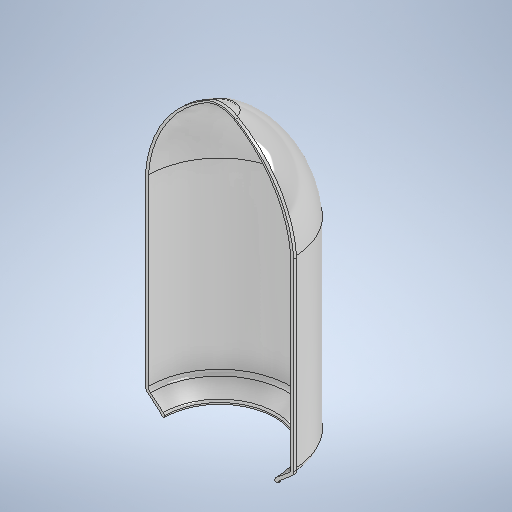
# Autodesk Inventor part: PAY-LOAD
Saved by Autodesk Inventor 2025 (Build 290162000, 162)
## iProperties
Created: 2024-07-25
Part Number: PAY-LOAD
Material: Generic
Document SubType Name: Modeling
Designer: Richard
Density: 1 g/cm^3
Appearance: Default
Author: Richard
Autodesk Inventor part; units mm, degrees
ref_plane "YZ Plane" through (0, 0, 0) normal (1, 0, 0) x (0, 1, 0)
ref_plane "XZ Plane" through (0, 0, 0) normal (0, 1, 0) x (-1, 0, 0)
ref_plane "XY Plane" through (0, 0, 0) normal (0, 0, 1) x (1, 0, 0)
sketch "Sketch1" plane through (0, 0, 0) normal (0, 0, 1) x (1, 0, 0)
  line L0 (0, 0) -> (39, 0)
  line L1 (0, 0.6011) -> (0, 0)
  line L2 (1, 1.0674) -> (1, 0)
  line L3 (39, 2) -> (39, 202)
  line L4 (-10, 138.8438) -> (-10, 13.0953)
  line L5 (0.2856, 2.5995) -> (-8.5712, 10.0311)
  line L6 (1, 2) -> (17.3022, 2) construction
  line L7 (0, 2) -> (16.6045, 2) construction
  line L8 (-6.0027, 6.5705) -> (-0.7144, 2.1332)
  line L9 (-6.0027, 6.5705) -> (-9.5712, 9.5648)
  line L10 (-11, 138.8438) -> (-11, 12.629)
  arc A0 (-10, 13.0953) -> (-8.5712, 10.0311) centre (-6, 13.0953) ccw
  arc A1 (-11, 12.629) -> (-9.5712, 9.5648) centre (-7, 12.629) ccw
  arc A2 (29, 202) -> (-11, 138.8438) centre (68.7541, 132.5766) ccw
  arc A3 (30, 202) -> (-10, 138.8438) centre (69.7541, 132.5766) ccw
  line L11 (39, 204.4115) -> (39, 205.0334)
  line L12 (39, 2) -> (39, 0)
  arc A4 (1, 1.0674) -> (0.2856, 2.5995) centre (-1, 1.0674) ccw
  arc A5 (0, 0.6011) -> (-0.7144, 2.1332) centre (-2, 0.6011) ccw
  line L13 (0, 0) -> (-1, 0)
  line L14 (-5.4284, 4.7832) -> (-10.5712, 9.0985)
  line L15 (-5.4284, 4.7832) -> (-1.7144, 1.6669)
  line L16 (-1, 0) -> (-1, 0.1348)
  line L17 (-11, 138.8438) -> (-12, 138.8438)
  line L18 (-12, 138.8438) -> (-12, 12.1627)
  arc A6 (-12, 12.1627) -> (-10.5712, 9.0985) centre (-8, 12.1627) ccw
  arc A7 (-1, 0.1348) -> (-1.7144, 1.6669) centre (-3, 0.1348) ccw
  arc A8 (28, 202) -> (-12, 138.8438) centre (67.7541, 132.5766) ccw
  arc A9 (39, 205.2967) -> (28, 202) centre (39, 185.2967) ccw
  arc A10 (39, 204.6795) -> (29, 202) centre (39, 184.6795) ccw
  arc A11 (39, 204.1394) -> (30, 202) centre (39, 184.1394) ccw
  line L19 (39, 204.1394) -> (39, 205.2967)
  line L20 (78, 0.6011) -> (78, 0)
  line L21 (84.0027, 6.5705) -> (78.7144, 2.1332)
  line L22 (84.0027, 6.5705) -> (87.5712, 9.5648)
  line L23 (89, 138.8438) -> (89, 12.629)
  arc A12 (87.5712, 9.5648) -> (89, 12.629) centre (85, 12.629) ccw
  arc A13 (89, 138.8438) -> (49, 202) centre (9.2459, 132.5766) ccw
  arc A14 (78.7144, 2.1332) -> (78, 0.6011) centre (80, 0.6011) ccw
  line L24 (78, 0) -> (79, 0)
  line L25 (83.4284, 4.7832) -> (88.5712, 9.0985)
  line L26 (83.4284, 4.7832) -> (79.7144, 1.6669)
  line L27 (90, 138.8438) -> (90, 12.1627)
  arc A15 (88.5712, 9.0985) -> (90, 12.1627) centre (86, 12.1627) ccw
  arc A16 (79.7144, 1.6669) -> (79, 0.1348) centre (81, 0.1348) ccw
  arc A17 (90, 138.8438) -> (50, 202) centre (10.2459, 132.5766) ccw
  arc A18 (50, 202) -> (39, 205.2967) centre (39, 185.2967) ccw
  arc A19 (49, 202) -> (39, 204.6795) centre (39, 184.6795) ccw
  dimension "d4" = 39
  dimension "d5" = 38
  dimension "d8" = 140
  dimension "d13" = 4
  dimension "d14" = 4
  dimension "d15" = 10
  dimension "d16" = 80
  dimension "d17" = 1
  dimension "d18" = 80
  dimension "d23" = 2
  dimension "d24" = 1
  dimension "d26" = 1
  dimension "d27" = 4
  dimension "d28" = 2
  dimension "d29" = 1
  dimension "d30" = 80
  dimension "d32" = 20
  dimension "d35" = 20
  dimension "d36" = 20
  constraints: 56 end point, 40 point on circle, 22 symmetric about line, 20 centre point, 12 tangent, 5 horizontal, 4 point on line, 2 parallel, 2 perpendicular, 2 vertical, 1 equal radius, 8 other
  measures "d4" distance of L3.start L7.start
  measures "d5" distance of L3.start L6.start
  measures "d8" angle of L6 L5
  measures "d13" radius of A0
  measures "d14" radius of A1
  measures "d15" distance of L3.end A2.start
  measures "d16" radius of A2
  measures "d17" distance of A2.start A3.start
  measures "d18" radius of A3
  measures "d23" radius of A4
  measures "d24" distance of L0.start L13.end
  measures "d26" distance of L10.start L17.end
  measures "d27" radius of A6
  measures "d28" radius of A7
  measures "d29" distance of A2.start A8.start
  measures "d30" radius of A8
  measures "d32" radius of A9
  measures "d35" radius of A10
  measures "d36" radius of A11
revolve "Revolution1" add sketch "Sketch1" angle 180 about axis through (39, 2, 0) along (0, -1, 0) contours L1 A5 L8 L9 A1 L10 A2 A10 L11 L19 A11 A3 L4 A0 L5 A4 L2 L0
sketch "Sketch2" plane through (39, 184.6795, 0) normal (0, 0, 1) x (1, 0, 0)
  line L0 (-39, -184.6795) -> (-40, -184.6795)
  line L1 (-38.7144, -182.08) -> (-47.5712, -174.6483) projected
  line L2 (-42.8737, -178.59) -> (-44.4058, -177.3044)
  line L3 (-45.6914, -178.8365) -> (-40.7144, -183.0126)
  line L4 (-40.7144, -183.0126) -> (-49.5712, -175.581)
  line L5 (-40, -184.6795) -> (-40, -184.5447)
  line L6 (-51, -45.8357) -> (-51, -172.5168)
  arc A0 (11, 17.3205) -> (-11, 17.3205) centre (0, 0.6172) ccw
  arc A1 (-11, 17.3205) -> (-51, -45.8357) centre (28.7541, -52.1029) ccw
  arc A2 (-40, -184.5447) -> (-40.7144, -183.0126) centre (-42, -184.5447) ccw
  arc A3 (-51, -172.5168) -> (-49.5712, -175.581) centre (-47, -172.5168) ccw
  line L7 (-39, -184.6795) -> (39, -184.6795) projected
  line L8 (0, -184.6795) -> (0, -174.6483)
  line L9 (-47.5712, -174.6483) -> (47.5712, -174.6483) projected
  line L10 (39, -184.6795) -> (40, -184.6795)
  line L11 (40.7144, -183.0126) -> (49.5712, -175.581)
  arc A4 (40.7144, -183.0126) -> (40, -184.5447) centre (42, -184.5447) ccw
  arc A5 (49.5712, -175.581) -> (51, -172.5168) centre (47, -172.5168) ccw
  line L12 (40, -184.6795) -> (40, -184.5447)
  line L13 (51, -45.8357) -> (51, -172.5168)
  arc A6 (51, -45.8357) -> (11, 17.3205) centre (-28.7541, -52.1029) ccw
  line L14 (-50, -172.0505) -> (50, -172.0505) projected
  arc A7 (-10, 17.3205) -> (-50, -45.8357) centre (29.7541, -52.1029) ccw
  line L15 (40, -184.6795) -> (38, -184.6795)
  arc A8 (38.7144, -182.08) -> (38, -183.6121) centre (40, -183.6121) ccw projected
  line L16 (38, -183.6121) -> (38, -184.6795)
  line L17 (38.7144, -182.08) -> (47.5712, -174.6483)
  arc A9 (38.7144, -182.08) -> (38, -183.6121) centre (40, -183.6121) ccw
  line L18 (49, -45.8357) -> (49, -171.5842) projected
  line L19 (49, -171.5842) -> (49, -45.8357)
  arc A10 (47.5712, -174.6483) -> (49, -171.5842) centre (45, -171.5842) ccw projected
  arc A11 (47.5712, -174.6483) -> (49, -171.5842) centre (45, -171.5842) ccw
  line L20 (10, 17.3205) -> (9, 17.3205)
  arc A12 (49, -45.8357) -> (9, 17.3205) centre (-30.7541, -52.1029) ccw
  arc A13 (9, 17.3205) -> (-9, 17.3205) centre (0, -0.5401) ccw
  arc A14 (-9, 17.3205) -> (-49, -45.8357) centre (30.7541, -52.1029) ccw
  line L21 (-49, -171.5842) -> (-49, -45.8357) projected
  line L22 (-49, -45.8357) -> (-49, -171.5842)
  line L23 (-47.5712, -174.6483) -> (-38.7144, -182.08)
  line L24 (-39, -184.6795) -> (-38, -184.6795)
  line L25 (-38, -184.6795) -> (-38, -183.6121)
  arc A15 (-38, -183.6121) -> (-38.7144, -182.08) centre (-40, -183.6121) ccw
  arc A16 (-49, -171.5842) -> (-47.5712, -174.6483) centre (-45, -171.5842) ccw
  point P0 (48.5712, -175.1147)
  dimension "d38" = 1
  dimension "d43" = 1
  dimension "d44" = 1
  dimension "d45" = 20
  dimension "d46" = 80
  dimension "d47" = 2
  dimension "d48" = 4
  dimension "d49" = 80
  dimension "d52" = 80
  dimension "d57" = 2
  dimension "d58" = 4
  dimension "d59" = 1
  dimension "d60" = 80
  dimension "d61" = 20
  dimension "d62" = 1
  dimension "d63" = 20
  dimension "d64" = 2
  dimension "d65" = 80
  dimension "d66" = 1
  dimension "d67" = 2
  dimension "d68" = 4
  constraints: 40 end point, 30 point on circle, 15 centre point, 14 tangent, 11 point on line, 8 symmetric about line, 3 perpendicular, 2 midpoint, 2 parallel, 2 vertical, 1 collinear, 1 horizontal, 2 other
  measures "d38" distance of L0.start L0.end
  measures "d43" distance of A7.start A0.end
  measures "d44" distance of L20.start A0.start
  measures "d45" radius of A0
  measures "d46" radius of A1
  measures "d47" radius of A2
  measures "d48" radius of A3
  measures "d49" radius of A6
  measures "d52" radius of A7
  measures "d57" radius of A9
  measures "d58" radius of A11
  measures "d59" distance of L20.start L20.end
  measures "d60" radius of A12
  measures "d61" distance of L20.end A0.end
  measures "d62" distance of A7.start A13.end
  measures "d63" radius of A13
  measures "d64" distance of L6.start L21.end
  measures "d65" radius of A14
  measures "d66" distance of L0.start L24.end
  measures "d67" radius of A15
  measures "d68" radius of A16
extrude "Extrusion1" add sketch "Sketch2" against normal blind 2 contours L0 L5 A2 L3 L4 A3 L6 A1 A0 A6 L13 A5 L11 A4 L12 L10 L7 L16 A8 L17 A10 L18 A12 A13 A14 L21 A16 L1 A15 L25
body "Solid1"
